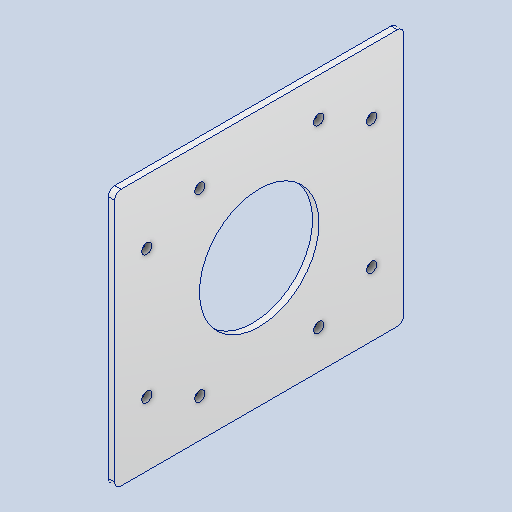
# Autodesk Inventor part: base_weel-v2-Plate-1
Saved by Autodesk Inventor 2025.2 (Build 292293000, 293)
## iProperties
Created: 2025-01-06
Part Number: base_weel-v2-Plate-1
Material: アルミニウム 6061
Document SubType Name: Modeling
Designer: haruy
Density: 2.7 g/cm^3
Appearance: アルミニウム - フラット
Mass: 32.9212 g
Surface Area: 131.809 cm^2
Volume: 12.193 cm^3
Author: haruy
Autodesk Inventor part; units mm, degrees
ref_plane "YZ Plane" through (0, 0, 0) normal (1, 0, 0) x (0, 1, 0)
ref_plane "XZ Plane" through (0, 0, 0) normal (0, 1, 0) x (-1, 0, 0)
ref_plane "XY Plane" through (0, 0, 0) normal (0, 0, 1) x (1, 0, 0)
derived "base_weel-v2-Sketch-Base.ipt"
ref_plane "作業平面1" through (0, 0, 0) normal (1, 0, 0) x (0, 1, 0)
sketch "スケッチ1" plane through (0, 0, 0) normal (1, 0, 0) x (0, 1, 0)
  line L0 (-315, 315) -> (315, 315) projected
  line L1 (315, 315) -> (315, -315) projected
  line L2 (315, -315) -> (-315, -315) projected
  line L3 (-315, -315) -> (-315, 315) projected
  line L4 (-315, 315) -> (315, -315) construction
  line L5 (315, 315) -> (-315, -315) construction
  line L6 (-295, 218) -> (-295, -202) projected
  line L7 (-295, -202) -> (-315, -202) projected
  line L8 (-315, -202) -> (-315, 210) projected
  line L9 (242, 315) -> (-242, 315) projected
  line L10 (-242, 315) -> (-242, 295) projected
  line L11 (-242, 295) -> (242, 295) projected
  line L12 (242, 295) -> (242, 315) projected
  line L13 (-295, 218) -> (-295, 315) projected
  line L14 (0, 0) -> (-956.5973, 0) projected
  circle A0 centre (0, 0) radius 400 projected
  line L15 (-330, 25) -> (-380, 25) projected
  line L16 (-380, 25) -> (-380, -25) projected
  line L17 (-380, -25) -> (-330, -25) projected
  line L18 (-330, -25) -> (-330, 25) projected
  line L19 (0, 0) -> (0, -630.9179) projected
  line L20 (-315, 40) -> (-395, 40) projected
  line L21 (-395, 40) -> (-395, 30) projected
  line L22 (-395, 30) -> (-315, 30) projected
  line L23 (-315, 30) -> (-315, 40) projected
  line L24 (-395, 30) -> (-385, 30) projected
  line L25 (-385, 30) -> (-385, 0) projected
  line L26 (-385, 0) -> (-395, 0) projected
  line L27 (-395, 0) -> (-395, 30) projected
  line L28 (295, 202) -> (315, 202) projected
  line L29 (315, 202) -> (315, -202) projected
  line L30 (315, -202) -> (295, -202) projected
  line L31 (295, -202) -> (295, 202) projected
  line L32 (-222.2183, -315) -> (242, -315) projected
  line L33 (242, -315) -> (242, -295) projected
  line L34 (242, -295) -> (-242, -295) projected
  line L35 (315, 315) -> (0, 0) construction
  line L36 (315, 125) -> (315, 145) projected
  circle A1 centre (512, 0) radius 122.5 projected
  circle A2 centre (179.6905, 0) radius 600 projected
  circle A3 centre (541.6815, 0) radius 200 projected
  circle A4 centre (0, 0) radius 10 construction
  arc A5 (0, 150) -> (0, -150) centre (0, 0) ccw projected
  arc A6 (0, 140) -> (0, -140) centre (0, 0) ccw projected
  line L37 (-146.3272, 32.9904) -> (-136.572, 30.791) projected
  line L38 (-137.5812, 37.6817) -> (-140.4404, 25) projected
  line L39 (-140.4404, 25) -> (-145.318, 26.0997) projected
  line L40 (-145.318, 26.0997) -> (-142.4588, 38.7814) projected
  line L41 (-142.4588, 38.7814) -> (-137.5812, 37.6817) projected
  arc A7 (-29.1302, 142.0438) -> (-29.1302, -142.0438) centre (0, 0) ccw projected
  circle A8 centre (-151.4904, 39.2799) radius 6.5 projected
  circle A9 centre (-129.0401, 34.2184) radius 6.5 construction
  circle A10 centre (-129.0401, 34.2184) radius 1.5 construction
  circle A11 centre (-151.4904, 39.2799) radius 1.5 projected
  line L42 (-30.1668, 22.5) -> (-174.1362, 22.5) construction
  line L43 (-174.1362, 22.5) -> (-174.1362, 7.5) projected
  line L44 (-174.1362, 7.5) -> (-30.1668, 7.5) construction
  line L45 (-30.1668, 7.5) -> (-30.1668, 22.5) construction
  circle A12 centre (-129.0401, -34.2184) radius 6.5 construction
  circle A13 centre (-129.0401, -34.2184) radius 1.5 construction
  line L46 (-142.4588, -38.7814) -> (-137.5812, -37.6817) projected
  line L47 (-145.318, -26.0997) -> (-142.4588, -38.7814) projected
  line L48 (-137.5812, -37.6817) -> (-140.4404, -25) projected
  line L49 (-140.4404, -25) -> (-145.318, -26.0997) projected
  circle A14 centre (-151.4904, -39.2799) radius 6.5 projected
  circle A15 centre (-151.4904, -39.2799) radius 1.5 projected
  line L50 (-146.3272, -32.9904) -> (-136.572, -30.791) projected
  line L51 (-30.1668, -22.5) -> (-174.1362, -22.5) construction
  line L52 (-174.1362, -7.5) -> (-30.1668, -7.5) construction
  line L53 (-30.1668, -7.5) -> (-30.1668, -22.5) construction
  line L54 (-174.1362, -22.5) -> (-174.1362, -7.5) projected
  line L55 (-151.4904, 39.2799) -> (-129.0401, 34.2184) construction
  line L56 (-129.0401, 34.2184) -> (-129.59, 31.7796) construction
  line L57 (-129.59, 31.7796) -> (-152.0402, 36.8412) construction
  line L58 (-152.0402, 36.8412) -> (-151.4904, 39.2799) construction
  line L59 (-129.0401, 34.2184) -> (-151.4904, 39.2799) construction
  line L60 (-151.4904, 39.2799) -> (-150.9405, 41.7187) construction
  line L61 (-150.9405, 41.7187) -> (-128.4903, 36.6572) construction
  line L62 (-128.4903, 36.6572) -> (-129.0401, 34.2184) construction
  line L63 (-128.4903, 36.6572) -> (-129.59, 31.7796) construction
  line L64 (-129.59, 31.7796) -> (-117.8838, 29.1404) construction
  line L65 (-117.8838, 29.1404) -> (-116.7841, 34.0179) construction
  line L66 (-116.7841, 34.0179) -> (-128.4903, 36.6572) construction
  line L67 (-150.9405, 41.7187) -> (-152.0402, 36.8412) construction
  line L68 (-152.0402, 36.8412) -> (-163.7464, 39.4804) construction
  line L69 (-163.7464, 39.4804) -> (-162.6467, 44.358) construction
  line L70 (-162.6467, 44.358) -> (-150.9405, 41.7187) construction
  line L71 (-155.2683, 45.2572) -> (-128.9412, 39.3216) projected
  line L72 (-128.9412, 39.3216) -> (-132.2403, 24.6889) projected
  line L73 (-132.2403, 24.6889) -> (-158.5673, 30.6245) projected
  line L74 (-158.5673, 30.6245) -> (-155.2683, 45.2572) projected
  line L75 (-128.9412, -39.3216) -> (-132.2403, -24.6889) projected
  line L76 (-155.2683, -45.2572) -> (-128.9412, -39.3216) projected
  line L77 (-132.2403, -24.6889) -> (-158.5673, -30.6245) projected
  line L78 (-158.5673, -30.6245) -> (-155.2683, -45.2572) projected
  arc A16 (-132.2403, 24.6889) -> (-132.2403, -24.6889) centre (0, 0) ccw projected
  arc A17 (-158.5673, 30.6245) -> (-158.5673, -30.6245) centre (0, 0) ccw projected
  circle A18 centre (-152.5, 15) radius 1.25 projected
  line L79 (-145, 0) -> (-145, 74.7382) projected
  circle A19 centre (-137.5, 15) radius 1.25 projected
  circle A20 centre (-137.5, -15) radius 1.25 projected
  circle A21 centre (-152.5, -15) radius 1.25 projected
  line L80 (0, 0) -> (0, 140) projected
  line L81 (0, 0) -> (-47.8828, 131.557) construction
  line L82 (0, 140) -> (0, 150) projected
  line L83 (-137.5846, 25.8938) -> (-134.2855, 40.5265) projected
  line L84 (-137.5846, -25.8938) -> (-134.2855, -40.5265) projected
  circle A22 centre (0, 0) radius 20 construction
  line L85 (295, 45) -> (-295, 45) projected
  line L86 (-295, 45) -> (-295, 25) projected
  line L87 (-295, 25) -> (295, 25) projected
  line L88 (295, 25) -> (295, 45) projected
  line L89 (-40, 295) -> (-50, 295) projected
  line L90 (-50, 295) -> (-50, 45) projected
  line L91 (-50, 45) -> (-40, 45) projected
  line L92 (-40, 45) -> (-40, 295) projected
  line L93 (-50, -295) -> (-50, -45) projected
  line L94 (-40, -45) -> (-40, -295) projected
  line L95 (295, -45) -> (-295, -45) projected
  line L96 (-295, -25) -> (295, -25) projected
  line L97 (-40, 45) -> (-40, -45) projected
  line L98 (40, 45) -> (40, -45) projected
  circle A23 centre (20, 35) radius 1.5 construction
  circle A24 centre (-20, 35) radius 1.5 construction
  circle A25 centre (-20, -35) radius 1.5 construction
  circle A26 centre (20, -35) radius 1.5 construction
  circle A27 centre (-45, 125) radius 1.5 projected
  circle A28 centre (-45, 125) radius 5 projected
  circle A29 centre (-130, 35) radius 5 projected
  circle A30 centre (-130, 35) radius 1.5 projected
  line L99 (-40, 134.1641) -> (-40, 125) projected
  line L100 (-50, 125) -> (-50, 130.767) projected
  line L101 (-137.7498, 25) -> (-127.5801, 30.6246) projected
  line L102 (-132.5707, 45) -> (-126.366, 38.4342) projected
  line L103 (-40, -134.1641) -> (-40, -125) projected
  circle A31 centre (-45, -125) radius 5 projected
  circle A32 centre (-45, -125) radius 1.5 projected
  line L104 (-50, -125) -> (-50, -130.767) projected
  line L105 (-132.5707, -45) -> (-126.366, -38.4342) projected
  circle A33 centre (-130, -35) radius 5 projected
  circle A34 centre (-130, -35) radius 1.5 projected
  line L106 (-137.7498, -25) -> (-127.5801, -30.6246) projected
  circle A35 centre (0, 0) radius 18.6
  line L107 (-242, -295) -> (-242, -315) projected
  line L108 (242, 315) -> (222, 315) projected
  line L109 (222, 315) -> (222, 295) projected
  line L110 (222, 295) -> (242, 295) projected
  line L111 (242, 295) -> (242, 315) projected
  line L112 (242, -315) -> (222, -315) projected
  line L113 (222, -315) -> (222, -295) projected
  line L114 (222, -295) -> (242, -295) projected
  line L115 (242, -295) -> (242, -315) projected
  line L116 (197, 295) -> (295, 197) projected
  line L117 (295, 197) -> (284.3934, 186.3934) projected
  line L118 (284.3934, 186.3934) -> (186.3934, 284.3934) projected
  line L119 (186.3934, 284.3934) -> (197, 295) projected
  line L120 (197, 295) -> (197, 315) projected
  line L121 (197.9167, 294.0833) -> (187.3101, 283.4767) projected
  line L122 (198.2703, 272.5165) -> (272.5165, 198.2703) projected
  line L123 (272.5165, 198.2703) -> (231.5043, 157.2581) projected
  line L124 (231.5043, 157.2581) -> (157.2581, 231.5043) projected
  line L125 (157.2581, 231.5043) -> (198.2703, 272.5165) projected
  line L126 (290.9013, 201.0987) -> (280.2947, 190.4921) projected
  line L127 (93.7624, 295) -> (295, 93.7624) projected
  line L128 (295, 93.7624) -> (284.3934, 83.1558) projected
  line L129 (284.3934, 83.1558) -> (83.1558, 284.3934) projected
  line L130 (214.1802, 277.8198) -> (203.5736, 267.2132) projected
  line L131 (277.8198, 214.1802) -> (267.2132, 203.5736) projected
  circle A36 centre (199.6845, 281.7089) radius 1.5 projected
  circle A37 centre (213.8266, 267.5668) radius 1.5 projected
  line L132 (186.3934, 284.3934) -> (175.7868, 295) projected
  circle A38 centre (187, 305) radius 1.5 projected
  circle A39 centre (177, 305) radius 1.5 projected
  line L133 (172, 315) -> (172, 295) projected
  line L134 (93.7624, 295) -> (93.7624, 295) projected
  line L135 (93.7624, 295) -> (93.7624, 315) projected
  line L136 (83.1558, 284.3934) -> (72.5492, 295) projected
  line L137 (68.7624, 315) -> (68.7624, 295) projected
  line L138 (284.3934, 186.3934) -> (295, 175.7868) projected
  line L139 (295, 197) -> (315, 197) projected
  line L140 (295, 93.7624) -> (295, 93.7624) projected
  line L141 (284.3934, 83.1558) -> (295, 72.5492) projected
  line L142 (-197, 295) -> (-197, 315) projected
  line L143 (-172, 315) -> (-172, 295) projected
  line L144 (-93.7624, 295) -> (-93.7624, 315) projected
  line L145 (-68.7624, 315) -> (-68.7624, 295) projected
  line L146 (-83.1558, 284.3934) -> (-72.5492, 295) projected
  line L147 (-93.7624, 295) -> (-295, 93.7624) projected
  line L148 (-83.1558, 284.3934) -> (-93.7624, 295) projected
  line L149 (-284.3934, 83.1558) -> (-83.1558, 284.3934) projected
  line L150 (-295, 93.7624) -> (-284.3934, 83.1558) projected
  line L151 (-284.3934, 83.1558) -> (-295, 72.5492) projected
  line L152 (-272.5165, 198.2703) -> (-231.5043, 157.2581) projected
  line L153 (-157.2581, 231.5043) -> (-198.2703, 272.5165) projected
  line L154 (-284.3934, 186.3934) -> (-186.3934, 284.3934) projected
  line L155 (-186.3934, 284.3934) -> (-175.7868, 295) projected
  line L156 (-197, 295) -> (-295, 197) projected
  line L157 (-197.9167, 294.0833) -> (-187.3101, 283.4767) projected
  line L158 (-214.1802, 277.8198) -> (-203.5736, 267.2132) projected
  line L159 (-290.9013, 201.0987) -> (-280.2947, 190.4921) projected
  line L160 (-284.3934, 186.3934) -> (-295, 175.7868) projected
  line L161 (-295, 197) -> (-315, 197) projected
  line L162 (-93.7624, -295) -> (-295, -93.7624) projected
  line L163 (-284.3934, -83.1558) -> (-83.1558, -284.3934) projected
  line L164 (-295, -93.7624) -> (-284.3934, -83.1558) projected
  line L165 (-197, -295) -> (-295, -197) projected
  line L166 (-284.3934, -186.3934) -> (-186.3934, -284.3934) projected
  line L167 (-290.9013, -201.0987) -> (-280.2947, -190.4921) projected
  line L168 (-214.1802, -277.8198) -> (-203.5736, -267.2132) projected
  line L169 (-197.9167, -294.0833) -> (-187.3101, -283.4767) projected
  line L170 (-83.1558, -284.3934) -> (-93.7624, -295) projected
  line L171 (284.3934, -83.1558) -> (83.1558, -284.3934) projected
  line L172 (83.1558, -284.3934) -> (93.7624, -295) projected
  line L173 (93.7624, -295) -> (295, -93.7624) projected
  line L174 (284.3934, -186.3934) -> (186.3934, -284.3934) projected
  line L175 (197.9167, -294.0833) -> (187.3101, -283.4767) projected
  line L176 (197, -295) -> (295, -197) projected
  line L177 (290.9013, -201.0987) -> (280.2947, -190.4921) projected
  line L178 (295, -93.7624) -> (284.3934, -83.1558) projected
  line L179 (242, 295) -> (222, 295) projected
  arc A40 (0, 86) -> (0, -86) centre (0, 0) ccw projected
  circle A41 centre (-90.8667, 48.5) radius 21 projected
  circle A42 centre (0, 0) radius 124 projected
  circle A43 centre (-90.8667, 48.5) radius 17 projected
  arc A44 (40.4951, 75.8693) -> (0, 86) centre (0, 0) ccw projected
  line L180 (-40, 45) -> (-50, 45) projected
  line L181 (-50, 45) -> (-50, -45) projected
  line L182 (-50, -45) -> (-40, -45) projected
  line L183 (-40, -45) -> (-40, 45) projected
  line L184 (-40, 295) -> (-50, 295) projected
  line L185 (-50, 295) -> (-50, 315) projected
  line L186 (-50, 315) -> (-40, 315) projected
  line L187 (-40, 315) -> (-40, 295) projected
  line L188 (-40, -295) -> (-50, -295) projected
  line L189 (-50, -295) -> (-50, -315) projected
  line L190 (-50, -315) -> (-40, -315) projected
  line L191 (-40, -315) -> (-40, -295) projected
  line L192 (40, -315) -> (40, -295) projected
  line L193 (50, -295) -> (50, -315) projected
  line L194 (50, -295) -> (50, -45) projected
  line L195 (40, -45) -> (40, -295) projected
  line L196 (40, -45) -> (40, 45) projected
  line L197 (50, 45) -> (50, -45) projected
  line L198 (40, 45) -> (40, 295) projected
  line L199 (50, 295) -> (50, 45) projected
  line L200 (40, 315) -> (40, 295) projected
  line L201 (50, 295) -> (50, 315) projected
  line L202 (-40.4092, 123.019) -> (-35, 135.5544) projected
  line L203 (-48.7417, 121.6834) -> (-55, 128.7439) projected
  line L204 (-40.4092, -123.019) -> (-35, -135.5544) projected
  line L205 (-48.7417, -121.6834) -> (-55, -128.7439) projected
  arc A45 (40.4951, 75.8693) -> (-40.4951, -75.8693) centre (0, 0) ccw projected
  circle A46 centre (0, 0) radius 86 construction
  circle A47 centre (0, 0) radius 78.5 projected
  circle A48 centre (-45, 58) radius 1.5 projected
  circle A49 centre (-45, 58) radius 5 projected
  circle A50 centre (45, 58) radius 5 projected
  circle A51 centre (45, 58) radius 1.5 projected
  line L206 (46.5549, 53.2479) -> (55, 56.0112) projected
  line L207 (40.325, 56.2267) -> (35, 70.2656) projected
  line L208 (50, 60.5165) -> (50, 69.9714) projected
  arc A52 (50, 69.9714) -> (40.4951, 75.8693) centre (0, 0) ccw projected
  line L209 (-40.325, 56.2267) -> (-35, 70.2656) projected
  line L210 (-46.5549, 53.2479) -> (-55, 56.0112) projected
  line L211 (-40.325, -56.2267) -> (-35, -70.2656) construction
  circle A53 centre (-45, -58) radius 5 projected
  line L212 (-46.5549, -53.2479) -> (-55, -56.0112) projected
  circle A54 centre (-45, -58) radius 1.5 projected
  line L213 (-40, -67.5444) -> (-40, -76.1315) projected
  arc A55 (-40.526, -75.8528) -> (-40, -76.1315) centre (0, 0) ccw projected
  line L214 (-40, -76.1315) -> (-40, -58) projected
  line L215 (222.6655, 269.3345) -> (212.0589, 258.7279) projected
  line L216 (269.3345, 222.6655) -> (258.7279, 212.0589) projected
  circle A56 centre (267.5668, 213.8266) radius 1.5 projected
  circle A57 centre (281.7089, 199.6845) radius 1.5 projected
  line L217 (294.0833, 197.9167) -> (283.4767, 187.3101) projected
  line L218 (315, 172) -> (295, 172) projected
  circle A58 centre (305, 177) radius 1.5 projected
  circle A59 centre (305, 187) radius 1.5 projected
  line L219 (295, 197) -> (315, 197) projected
  circle A60 centre (83.7624, 305) radius 1.5 projected
  circle A61 centre (73.7624, 305) radius 1.5 projected
  line L220 (197.9167, 294.0833) -> (94.6791, 294.0833) projected
  line L221 (187.3101, 283.4767) -> (84.0725, 283.4767) projected
  line L222 (94.6791, 294.0833) -> (84.0725, 283.4767) projected
  circle A62 centre (96.4469, 281.7089) radius 1.5 projected
  circle A63 centre (110.5891, 267.5668) radius 1.5 projected
  line L223 (119.4279, 269.3345) -> (108.8213, 258.7279) projected
  line L224 (295, 93.7624) -> (315, 93.7624) projected
  line L225 (315, 68.7624) -> (295, 68.7624) projected
  circle A64 centre (305, 73.7624) radius 1.5 projected
  circle A65 centre (305, 83.7624) radius 1.5 projected
  line L226 (294.0833, 94.6791) -> (283.4767, 84.0725) projected
  circle A66 centre (281.7089, 96.4469) radius 1.5 projected
  circle A67 centre (267.5668, 110.5891) radius 1.5 projected
  line L227 (269.3345, 119.4279) -> (258.7279, 108.8213) projected
  line L228 (-197, 295) -> (-197, 315) projected
  line L229 (-172, 315) -> (-172, 295) projected
  circle A68 centre (-177, 305) radius 1.5 projected
  circle A69 centre (-187, 305) radius 1.5 projected
  line L230 (-197.9167, 294.0833) -> (-187.3101, 283.4767) projected
  circle A70 centre (-199.6845, 281.7089) radius 1.5 projected
  line L231 (-214.1802, 277.8198) -> (-203.5736, 267.2132) projected
  circle A71 centre (-213.8266, 267.5668) radius 1.5 projected
  line L232 (-222.6655, 269.3345) -> (-212.0589, 258.7279) projected
  circle A72 centre (-267.5668, 213.8266) radius 1.5 projected
  line L233 (-269.3345, 222.6655) -> (-258.7279, 212.0589) projected
  circle A73 centre (-281.7089, 199.6845) radius 1.5 projected
  line L234 (-294.0833, 197.9167) -> (-283.4767, 187.3101) projected
  line L235 (-295, 197) -> (-315, 197) projected
  circle A74 centre (-305, 187) radius 1.5 projected
  circle A75 centre (-305, 177) radius 1.5 projected
  line L236 (-315, 172) -> (-295, 172) projected
  line L237 (-295, 93.7624) -> (-315, 93.7624) projected
  line L238 (-315, 68.7624) -> (-295, 68.7624) projected
  circle A76 centre (-305, 73.7624) radius 1.5 projected
  circle A77 centre (-305, 83.7624) radius 1.5 projected
  line L239 (-294.0833, 94.6791) -> (-283.4767, 84.0725) projected
  circle A78 centre (-281.7089, 96.4469) radius 1.5 projected
  circle A79 centre (-267.5668, 110.5891) radius 1.5 projected
  line L240 (-269.3345, 119.4279) -> (-258.7279, 108.8213) projected
  line L241 (-119.4279, 269.3345) -> (-108.8213, 258.7279) projected
  circle A80 centre (-110.5891, 267.5668) radius 1.5 projected
  circle A81 centre (-96.4469, 281.7089) radius 1.5 projected
  line L242 (-94.6791, 294.0833) -> (-84.0725, 283.4767) projected
  line L243 (-93.7624, 295) -> (-93.7624, 315) projected
  line L244 (-68.7624, 315) -> (-68.7624, 295) projected
  circle A82 centre (-73.7624, 305) radius 1.5 projected
  circle A83 centre (-83.7624, 305) radius 1.5 projected
  line L245 (-295, -197) -> (-315, -197) projected
  circle A84 centre (-305, -187) radius 1.5 projected
  circle A85 centre (-305, -177) radius 1.5 projected
  line L246 (-315, -172) -> (-295, -172) projected
  line L247 (-294.0833, -197.9167) -> (-283.4767, -187.3101) projected
  circle A86 centre (-281.7089, -199.6845) radius 1.5 projected
  circle A87 centre (-267.5668, -213.8266) radius 1.5 projected
  line L248 (-269.3345, -222.6655) -> (-258.7279, -212.0589) projected
  line L249 (-222.6655, -269.3345) -> (-212.0589, -258.7279) projected
  circle A88 centre (-213.8266, -267.5668) radius 1.5 projected
  circle A89 centre (-199.6845, -281.7089) radius 1.5 projected
  line L250 (-197.9167, -294.0833) -> (-187.3101, -283.4767) projected
  line L251 (-197, -295) -> (-197, -315) projected
  circle A90 centre (-187, -305) radius 1.5 projected
  circle A91 centre (-177, -305) radius 1.5 projected
  line L252 (-172, -315) -> (-172, -295) projected
  line L253 (-295, -93.7624) -> (-315, -93.7624) projected
  circle A92 centre (-305, -83.7624) radius 1.5 projected
  circle A93 centre (-305, -73.7624) radius 1.5 projected
  line L254 (-315, -68.7624) -> (-295, -68.7624) projected
  line L255 (-294.0833, -94.6791) -> (-283.4767, -84.0725) projected
  circle A94 centre (-281.7089, -96.4469) radius 1.5 projected
  circle A95 centre (-267.5668, -110.5891) radius 1.5 projected
  line L256 (-269.3345, -119.4279) -> (-258.7279, -108.8213) projected
  line L257 (-119.4279, -269.3345) -> (-108.8213, -258.7279) projected
  circle A96 centre (-110.5891, -267.5668) radius 1.5 projected
  circle A97 centre (-96.4469, -281.7089) radius 1.5 projected
  line L258 (-94.6791, -294.0833) -> (-84.0725, -283.4767) projected
  line L259 (-93.7624, -295) -> (-93.7624, -315) projected
  circle A98 centre (-83.7624, -305) radius 1.5 projected
  circle A99 centre (-73.7624, -305) radius 1.5 projected
  line L260 (-68.7624, -315) -> (-68.7624, -295) projected
  line L261 (68.7624, -315) -> (68.7624, -295) projected
  circle A100 centre (73.7624, -305) radius 1.5 projected
  circle A101 centre (83.7624, -305) radius 1.5 projected
  line L262 (93.7624, -295) -> (93.7624, -315) projected
  line L263 (94.6791, -294.0833) -> (84.0725, -283.4767) projected
  circle A102 centre (96.4469, -281.7089) radius 1.5 projected
  circle A103 centre (110.5891, -267.5668) radius 1.5 projected
  line L264 (119.4279, -269.3345) -> (108.8213, -258.7279) projected
  line L265 (172, -315) -> (172, -295) projected
  circle A104 centre (177, -305) radius 1.5 projected
  circle A105 centre (187, -305) radius 1.5 projected
  line L266 (197, -295) -> (197, -315) projected
  line L267 (197.9167, -294.0833) -> (187.3101, -283.4767) projected
  circle A106 centre (199.6845, -281.7089) radius 1.5 projected
  circle A107 centre (213.8266, -267.5668) radius 1.5 projected
  line L268 (222.6655, -269.3345) -> (212.0589, -258.7279) projected
  line L269 (269.3345, -222.6655) -> (258.7279, -212.0589) projected
  circle A108 centre (267.5668, -213.8266) radius 1.5 projected
  circle A109 centre (281.7089, -199.6845) radius 1.5 projected
  line L270 (294.0833, -197.9167) -> (283.4767, -187.3101) projected
  line L271 (295, -197) -> (315, -197) projected
  circle A110 centre (305, -187) radius 1.5 projected
  circle A111 centre (305, -177) radius 1.5 projected
  line L272 (315, -172) -> (295, -172) projected
  line L273 (295, -93.7624) -> (315, -93.7624) projected
  circle A112 centre (305, -83.7624) radius 1.5 projected
  circle A113 centre (305, -73.7624) radius 1.5 projected
  line L274 (315, -68.7624) -> (295, -68.7624) projected
  line L275 (294.0833, -94.6791) -> (283.4767, -84.0725) projected
  circle A114 centre (281.7089, -96.4469) radius 1.5 projected
  line L276 (269.3345, -119.4279) -> (258.7279, -108.8213) projected
  circle A115 centre (267.5668, -110.5891) radius 1.5 projected
  line L277 (-295, 202) -> (-315, 202) projected
  line L278 (265, 45) -> (265, 25) projected
  circle A116 centre (275, 35) radius 1.5 projected
  circle A117 centre (285, 35) radius 1.5 projected
  circle A118 centre (305, 35) radius 1.5 projected
  circle A119 centre (305, 25) radius 1.5 projected
  line L279 (295, 25) -> (315, 25) projected
  line L280 (265, -45) -> (265, -25) projected
  circle A120 centre (275, -35) radius 1.5 projected
  circle A121 centre (285, -35) radius 1.5 projected
  circle A122 centre (305, -35) radius 1.5 projected
  circle A123 centre (305, -25) radius 1.5 projected
  circle A124 centre (-305, -25) radius 1.5 projected
  circle A125 centre (-305, -35) radius 1.5 projected
  circle A126 centre (-285, -35) radius 1.5 projected
  circle A127 centre (-275, -35) radius 1.5 projected
  line L281 (-265, -45) -> (-265, -25) projected
  line L282 (-265, 45) -> (-265, 25) projected
  circle A128 centre (-275, 35) radius 1.5 projected
  circle A129 centre (-285, 35) radius 1.5 projected
  circle A130 centre (-305, 35) radius 1.5 projected
  circle A131 centre (-305, 25) radius 1.5 projected
  circle A132 centre (48, 345) radius 44 projected
  circle A133 centre (-50, 345) radius 44 projected
  circle A134 centre (-50, 345) radius 15 projected
  line L283 (295, 45) -> (315, 45) projected
  line L284 (295, 15) -> (315, 15) projected
  line L285 (-315, 45.5) -> (-390, 45.5) projected
  line L286 (-390, 45.5) -> (-390, 0) projected
  line L287 (-390, 0) -> (-315, 0) projected
  line L288 (-315, 0) -> (-315, 45.5) projected
  circle A135 centre (-305, 48) radius 1.5 projected
  circle A136 centre (-305, -48) radius 1.5 projected
  line L289 (114.7878, 210) -> (54.7878, 210) projected
  line L290 (54.7878, 210) -> (54.7878, 270) projected
  line L291 (54.7878, 270) -> (114.7878, 270) projected
  line L292 (114.7878, 270) -> (114.7878, 210) projected
  line L293 (34.7878, 210) -> (-25.2122, 210) projected
  line L294 (-25.2122, 210) -> (-25.2122, 270) projected
  line L295 (-25.2122, 270) -> (34.7878, 270) projected
  line L296 (34.7878, 270) -> (34.7878, 210) projected
  line L297 (-45.2122, 250) -> (-115.2122, 250) projected
  line L298 (-115.2122, 250) -> (-115.2122, 266) projected
  line L299 (-115.2122, 266) -> (-45.2122, 266) projected
  line L300 (-45.2122, 266) -> (-45.2122, 250) projected
  line L301 (-50.2122, 214) -> (-110.2122, 214) projected
  line L302 (-110.2122, 214) -> (-110.2122, 230) projected
  line L303 (-110.2122, 230) -> (-50.2122, 230) projected
  line L304 (-50.2122, 230) -> (-50.2122, 214) projected
  circle A137 centre (0, 0) radius 175.5 projected
  line L305 (-185, -89) -> (-302, -89) projected
  line L306 (-302, -89) -> (-302, 89) projected
  line L307 (-302, 89) -> (-185, 89) projected
  line L308 (-185, 89) -> (-185, -89) projected
  line L309 (287, -17.7878) -> (205, -17.7878) projected
  line L310 (205, -17.7878) -> (205, 79.2122) projected
  line L311 (205, 79.2122) -> (287, 79.2122) projected
  line L312 (287, 79.2122) -> (287, -17.7878) projected
  line L313 (284.5, -114.7878) -> (207.5, -114.7878) projected
  line L314 (207.5, -114.7878) -> (207.5, -37.7878) projected
  line L315 (207.5, -37.7878) -> (284.5, -37.7878) projected
  line L316 (284.5, -37.7878) -> (284.5, -114.7878) projected
  line L317 (281, 99.2122) -> (211, 99.2122) projected
  line L318 (211, 99.2122) -> (211, 115.2122) projected
  line L319 (211, 115.2122) -> (281, 115.2122) projected
  line L320 (281, 115.2122) -> (281, 99.2122) projected
  line L321 (137.7122, 315) -> (-137.7122, 315) projected
  line L322 (-137.7122, 315) -> (-137.7122, 185) projected
  line L323 (-137.7122, 185) -> (137.7122, 185) projected
  line L324 (137.7122, 185) -> (137.7122, 315) projected
  line L325 (315, -137.7122) -> (185, -137.7122) projected
  line L326 (185, -137.7122) -> (185, 137.7122) projected
  line L327 (185, 137.7122) -> (315, 137.7122) projected
  line L328 (315, 137.7122) -> (315, -137.7122) projected
  line L329 (258.7782, 137.7122) -> (278.7782, 137.7122) projected
  line L330 (278.7782, 137.7122) -> (278.7782, 127.7122) projected
  line L331 (278.7782, 127.7122) -> (258.7782, 127.7122) projected
  line L332 (258.7782, 127.7122) -> (258.7782, 137.7122) projected
  circle A138 centre (268.7782, 132.7122) radius 1.5 projected
  line L333 (278.7782, 137.7122) -> (231.1981, 137.7122) projected
  line L334 (231.1981, 137.7122) -> (231.1981, 147.7122) projected
  line L335 (231.1981, 147.7122) -> (278.7782, 147.7122) projected
  line L336 (278.7782, 147.7122) -> (278.7782, 137.7122) projected
  line L337 (255.1924, 112.3568) -> (233.9792, 133.57) projected
  line L338 (233.9792, 133.57) -> (230.4437, 130.0345) projected
  line L339 (230.4437, 130.0345) -> (251.6569, 108.8213) projected
  line L340 (251.6569, 108.8213) -> (255.1924, 112.3568) projected
  line L341 (288.78, 89.3758) -> (114.1246, 264.0312) projected
  line L342 (269.3345, 126.499) -> (265.799, 122.9634) projected
  line L343 (248.1213, 147.7122) -> (269.3345, 126.499) projected
  line L344 (244.5858, 144.1766) -> (248.1213, 147.7122) projected
  circle A139 centre (268.7782, 132.7122) radius 4 projected
  line L345 (233.9792, 133.57) -> (244.5858, 144.1766) projected
  line L346 (-330, 143.5) -> (-340, 143.5) projected
  line L347 (-340, 143.5) -> (-340, -143.5) projected
  line L348 (-340, -143.5) -> (-330, -143.5) projected
  line L349 (-330, -143.5) -> (-330, 143.5) projected
  line L350 (-315, 119) -> (-295, 119) projected
  line L351 (-295, 119) -> (-295, 104) projected
  line L352 (-295, 104) -> (-315, 104) projected
  line L353 (-315, 104) -> (-315, 119) projected
  line L354 (-315, 153.5) -> (-325, 153.5) projected
  line L355 (-325, 153.5) -> (-325, 0) projected
  line L356 (-325, 0) -> (-315, 0) projected
  line L357 (-315, 0) -> (-315, 153.5) projected
  line L358 (-340, 133.5) -> (-345, 133.5) projected
  line L359 (-345, 133.5) -> (-345, 143.5) projected
  line L360 (-345, 143.5) -> (-340, 143.5) projected
  line L361 (-340, 143.5) -> (-340, 133.5) projected
  line L362 (-330, 133.5) -> (-325, 133.5) projected
  line L363 (-325, 133.5) -> (-325, 143.5) projected
  line L364 (-325, 143.5) -> (-330, 143.5) projected
  line L365 (-330, 143.5) -> (-330, 133.5) projected
  line L366 (-325, 153.5) -> (-345, 153.5) projected
  line L367 (-345, 153.5) -> (-345, 143.5) projected
  line L368 (-345, 143.5) -> (-325, 143.5) projected
  line L369 (-325, 143.5) -> (-325, 153.5) projected
  line L370 (-295, 104) -> (-345, 104) projected
  line L371 (-345, 104) -> (-345, 98) projected
  line L372 (-345, 98) -> (-295, 98) projected
  line L373 (-295, 98) -> (-295, 104) projected
  line L374 (185, -25) -> (180, -25) projected
  line L375 (180, -25) -> (180, -15) projected
  line L376 (180, -15) -> (185, -15) projected
  line L377 (185, -15) -> (185, -25) projected
  line L378 (185, -25) -> (195, -25) projected
  line L379 (195, -25) -> (195, -15) projected
  line L380 (195, -15) -> (185, -15) projected
  line L381 (185, -15) -> (185, -25) projected
  line L382 (40, 180) -> (30, 180) projected
  line L383 (30, 180) -> (30, 195) projected
  line L384 (30, 195) -> (40, 195) projected
  line L385 (40, 195) -> (40, 180) projected
  circle A140 centre (-132.7122, 268.7782) radius 1.5 projected
  circle A141 centre (132.7122, 268.7782) radius 1.5 projected
  line L386 (-243.5, 89) -> (-243.5, -89) projected
  circle A142 centre (-214, 35) radius 1.5 projected
  circle A143 centre (-214, -35) radius 1.5 projected
  line L387 (-214, 89) -> (-214, -89) projected
  line L388 (-246, 89) -> (-246, -89) projected
  circle A144 centre (-254.5, 35) radius 4 projected
  circle A145 centre (-254.5, -35) radius 4 projected
  circle A146 centre (0, 0) radius 100 projected
  circle A147 centre (-134.1671, -14.9726) radius 5 projected
  circle A148 centre (-134.1671, -14.9726) radius 1.25 projected
  circle A149 centre (-134.9074, -5) radius 5 projected
  circle A150 centre (-134.9074, -5) radius 1.25 projected
  circle A151 centre (20, 35) radius 1.6
  circle A152 centre (-20, 35) radius 1.6
  circle A153 centre (-20, -35) radius 1.6
  circle A154 centre (20, -35) radius 1.6
  circle A155 centre (0, 0) radius 20 construction
  circle A156 centre (0, 0) radius 16 construction
  line L389 (-33, 21) -> (0, 21)
  line L390 (0, 21) -> (0, 16)
  line L391 (0, 16) -> (-33, 16)
  line L392 (-33, 16) -> (-33, 21)
  circle A157 centre (-28, 18.5) radius 1.6
  circle A158 centre (0, 0) radius 24 construction
  circle A159 centre (0, 0) radius 28 construction
  circle A160 centre (-28, 18.5) radius 4
  line L393 (33, 21) -> (0, 21)
  line L394 (0, 16) -> (33, 16)
  line L395 (33, 16) -> (33, 21)
  circle A161 centre (28, 18.5) radius 1.6
  line L396 (-33, -21) -> (0, -21)
  line L397 (0, -16) -> (-33, -16)
  line L398 (-33, -16) -> (-33, -21)
  circle A162 centre (-28, -18.5) radius 1.6
  line L399 (33, -21) -> (0, -21)
  line L400 (0, -16) -> (33, -16)
  circle A163 centre (28, -18.5) radius 1.6
  line L401 (33, -16) -> (33, -21)
  point P0 (-141.4496, 31.8907)
  point P1 (-129.0401, 34.2184)
  point P2 (-150, 0)
  point P3 (-40, 45)
  point P4 (-40, -45)
  point P5 (-242, 305)
  point P6 (-295, 93.7624)
  point P7 (-161.4975, 0)
  point P8 (305, 25)
  point P9 (295, 35)
  dimension "d1" = 37.2
  dimension "d5" = 3.2
  dimension "d6" = 3.2
  dimension "d7" = 3.2
  dimension "d8" = 3.2
  dimension "d9" = 40
  dimension "d10" = 32
  dimension "d11" = 5
  dimension "d12" = 3.2
  dimension "d13" = 5
  dimension "d14" = 2.5
  dimension "d16" = 48
  dimension "d17" = 4
  dimension "d18" = 8
  dimension "d19" = 28
  dimension "d20" = 0
  constraints: 26 end point, 14 centre point, 11 coincident, 11 symmetric about line, 2 parallel, 1 horizontal, 1 perpendicular, 1 tangent, 4 other
  measures "d1" diameter of A35
  measures "d5" diameter of A151
  measures "d6" diameter of A152
  measures "d7" diameter of A153
  measures "d8" diameter of A154
  measures "d9" diameter of A155
  measures "d10" diameter of A156
  measures "d11" distance between parallel lines of L389 L391
  measures "d12" diameter of A157
  measures "d13" distance from line of L392 A157.centre
  measures "d14" distance from line of L389 A157.centre
  measures "d16" diameter of A158
  measures "d17" radial gap between concentric circles of A158 A159
  measures "d18" diameter of A160
  measures "d19" distance from line of A160.centre L80
  measures "d20" distance between parallel lines of L80 L390
extrude "押し出し1" add sketch "スケッチ1" against normal blind 2 contours L95 L19 L96 L98 | L95 L97 L96 L19 | L96 L19 L399 L401 L400 A35 L394 L395 L393 L80 L87 L98 | L96 L97 L14 A35 L397 L398 L396 L19 | L87 L80 L85 L98 | L396 L398 L397 A35 L19 | L19 A35 L400 L401 L399 | L87 L97 L85 L80 | L80 L389 A160 L392 L391 A35 L14 L97 L87 | L393 L395 L394 A35 L80 | L80 A35 L391 A160 L389 | A160 L391 L389 | L389 A160 | A160 L391 L392 L389 | A160 L391
fillet "フィレット1" radius 2 4 edges at (-1, 40, 45) (-1, 40, -45) (-1, -40, -45) (-1, -40, 45)
